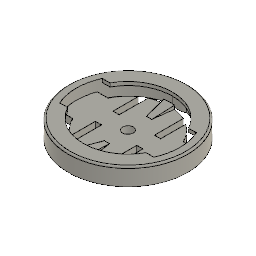
Blendr_Garmin_mount (Autodesk Fusion 360 design; units mm, degrees)
Autodesk Fusion 360 part; units mm, degrees
sketch "Sketch1" plane through (0, 0, 0) normal (0, 0, 1) x (1, 0, 0)
  circle A0 centre (0, 0) radius 1.5
  circle A1 centre (0, 0) radius 16.9
  circle A2 centre (0, 0) radius 14.6
  line L0 (0, 0) -> (25.4189, 0) construction
  line L1 (-6.75, -9.6177) -> (-6.75, 9.6177) construction
  line L2 (6.75, 9.6177) -> (6.75, -10.6368) construction
  line L3 (-6.75, 9.6177) -> (-6.75, 5)
  line L4 (6.75, 5) -> (6.75, 9.6177)
  line L5 (-6.75, -9.6177) -> (-6.75, -5)
  line L6 (6.75, -9.6177) -> (6.75, -5)
  line L7 (-10.6331, 5) -> (-13.7171, 5)
  line L8 (-13.7171, -5) -> (-10.6331, -5)
  arc A3 (-5, -10.6331) -> (5, -10.6331) centre (0, 0) ccw
  line L9 (13.7171, 5) -> (10.6331, 5)
  line L10 (10.6331, -5) -> (13.7171, -5)
  arc A4 (6.75, -9.6177) -> (10.6331, -5) centre (0, 0) ccw
  arc A5 (-6.75, 9.6177) -> (-10.6331, 5) centre (0, 0) ccw
  arc A6 (-10.6331, -5) -> (-6.75, -9.6177) centre (0, 0) ccw
  line L11 (-13.3404, 6) -> (-13.3404, -6) construction
  line L12 (13.3404, -6) -> (13.3404, 6) construction
  line L13 (-11.0797, 6) -> (-13.3404, 6)
  line L14 (11.0797, 6) -> (13.3404, 6)
  line L15 (13.3101, -6) -> (11.0797, -6)
  line L16 (-13.3101, -6) -> (-11.0797, -6)
  line L17 (-13.3404, -6) -> (-11.0797, -6) construction
  line L18 (-11.0797, 6) -> (-13.3404, 6) construction
  arc A7 (11.0797, 6) -> (-11.0797, 6) centre (0, 0) ccw
  line L19 (13.3404, 6) -> (11.0797, 6) construction
  line L20 (10.1026, 6) -> (-10.1026, 6) construction
  arc A8 (-11.0797, -6) -> (11.0797, -6) centre (0, 0) ccw
  line L21 (-10.1026, -6) -> (10.1026, -6) construction
  line L22 (11.0797, -6) -> (13.3404, -6) construction
  arc A9 (10.6331, 5) -> (6.75, 9.6177) centre (0, 0) ccw
  arc A10 (5, 10.6331) -> (-5, 10.6331) centre (0, 0) ccw
  line L23 (-5, -10.6368) -> (-5, -5)
  line L24 (-5, 5) -> (-5, 10.6368)
  line L25 (5, 10.6368) -> (5, 5)
  line L26 (5, -5) -> (5, -10.6368)
  line L27 (-5, 5) -> (-5, 2.5)
  line L28 (-5, 2.5) -> (-6.75, 2.5)
  line L29 (-6.75, 2.5) -> (-6.75, 5)
  line L30 (-5, -5) -> (-5, -2.5)
  line L31 (-5, -2.5) -> (-6.75, -2.5)
  line L32 (-6.75, -2.5) -> (-6.75, -5)
  line L33 (6.75, -5) -> (6.75, -2.5)
  line L34 (6.75, -2.5) -> (5, -2.5)
  line L35 (5, -2.5) -> (5, -5)
  line L36 (6.75, 5) -> (6.75, 2.5)
  line L37 (6.75, 2.5) -> (5, 2.5)
  line L38 (5, 2.5) -> (5, 5)
  line L39 (1.5, -11.75) -> (-1.5, -11.75) construction
  line L40 (-1.5, -11.75) -> (-1.5, 11.75) construction
  line L41 (-1.5, 11.75) -> (1.5, 11.75) construction
  line L42 (1.5, 11.75) -> (1.5, -11.75) construction
  line L43 (1.5, -11.75) -> (-1.5, 11.75) construction
  line L44 (-1.5, -11.75) -> (1.5, 11.75) construction
  arc A11 (-0.7598, -5.9517) -> (0.7598, -5.9517) centre (0, 0) ccw
  line L45 (-0.7598, -5.9517) -> (-1.4879, -11.6554)
  line L46 (0.7598, -5.9517) -> (1.5, -11.75)
  arc A12 (0.7598, 5.9517) -> (-0.7598, 5.9517) centre (0, 0) ccw
  line L47 (-0.7598, 5.9517) -> (-1.4879, 11.6554)
  line L48 (1.5, 11.6539) -> (0.7598, 5.9517)
  line L49 (0, 0) -> (0, 17.8654) construction
  line L50 (0, 0) -> (0, -17.7378) construction
  arc A13 (1.9907, -14.4637) -> (-1.9907, -14.4637) centre (0, -18.52) ccw
  arc A14 (-2.0011, 14.4622) -> (2.0011, 14.4622) centre (0, 18.5154) ccw
  dimension "d1" = 3
  dimension "d2" = 23.5
  dimension "d4" = 33.8
  dimension "d5" = 29.2
  dimension "d10" = 12
  dimension "d11" = 2.5
  dimension "d12" = 2.5
  dimension "d13" = 2.5
  dimension "d14" = 2.5
  dimension "d15" = 3
  dimension "d16" = 23.5
  dimension "d18" = 6
  dimension "d19" = 6
  constraint coincident A0.centre A1.centre
  constraint concentric A2 A5
  constraint horizontal L0
  constraint horizontal L9
  constraint parallel L8 L9
  constraint parallel L23 L25
  constraint parallel L1 L2
  constraint coincident L1 L3.end
  constraint coincident L2 L4.start
  constraint coincident L4.start L9
  constraint coincident L2.start A5
  constraint coincident L5.end L8
  constraint coincident L1 L5.end
  constraint coincident L6.start A5
  constraint coincident L2 L6.start
  constraint coincident L2 L6.end
  constraint coincident L6.end L8
  constraint coincident A10.end L23
  constraint collinear L7 L9
  constraint coincident L8.end A5
  constraint coincident A3.start L23
  constraint concentric A3 A5
  constraint coincident A3.end L25
  constraint concentric A3 A4
  constraint coincident L9.end A4
  constraint concentric A4 A9
  constraint concentric A5 A6
  constraint horizontal L19
  constraint perpendicular L11 L19
  constraint parallel L17 L19
  constraint parallel L11 L12
  constraint coincident L13.start L19
  constraint coincident L15.start L17
  constraint coincident A2 L15.start
  constraint coincident L15.end L17
  constraint coincident A2 L16.start
  constraint coincident L16.start L17
  constraint coincident A6 L21.start
  constraint collinear L17 L21
  constraint coincident A5 L20.end
  constraint collinear L18 L19
  constraint coincident L20.start A9
  constraint collinear L19 L20
  constraint coincident A4 L21.end
  constraint collinear L21 L22
  constraint coincident A10.start L25
  constraint concentric A9 A10
  constraint collinear L23 L24
  constraint collinear L25 L26
  constraint vertical L27
  constraint horizontal L28
  constraint vertical L29
  constraint vertical L30
  constraint horizontal L31
  constraint vertical L32
  constraint vertical L33
  constraint horizontal L34
  constraint vertical L35
  constraint vertical L36
  constraint horizontal L37
  constraint vertical L38
  constraint horizontal L39
  constraint perpendicular L39 L40
  constraint parallel L39 L41
  constraint parallel L40 L42
  constraint coincident L43 A0.centre
  constraint coincident L44 A0.centre
  constraint coincident L44 A11.start
  constraint coincident A3 L45.end
  constraint coincident L44 L45.end
  constraint parallel L43 L46
  constraint coincident L43 A12.end
  constraint coincident A10 L47.end
  constraint coincident L43 L47.end
  constraint coincident A10 L48.start
  constraint coincident L42 L48.start
  constraint coincident A2 L9.start
  constraint coincident A2 L10.end
  constraint coincident A2 L7.end
  constraint coincident A2 L8.start
  constraint vertical L49
  constraint vertical L50
  constraint coincident A2 A13.end
  constraint coincident A2 A13.start
  constraint coincident A2 A14.start
  constraint coincident A2 A14.end
  measures "d1" diameter of A0
  measures "d2" diameter of A5
  measures "d4" diameter of A1
  measures "d5" diameter of A2
  measures "d10" distance of L11.start L11.end
  measures "d11" distance of L3.end L28.end
  measures "d12" distance of L5.end L31.end
  measures "d13" distance of L26.start L34.end
  measures "d14" distance of L25.end L37.end
  measures "d15" distance of L40.end L41.end
  measures "d16" distance of L39.end L40.end
  measures "d18" radius of A11
  measures "d19" radius of A12
extrude "Extrude1" add sketch "Sketch1" along normal blind 2 contours A2 L3 L4 L5 L6 L7 L8 A3 L9 L10 A4 A5 A6 A9 A10 L23 L24 L25 L26 L27 L28 L29 L30 L31 L32 L33 L34 L35 L36 L37 L38 A11 L45 L46 A12 L47 L48
extrude "Extrude2" add sketch "Sketch1" along normal blind 3 contours A10 A12 L47 L48
chamfer "Chamfer1" distance 5.75 distance2 1 1 edges at (0, 6, 3) measured on face at (0.9217, 9.7816, 3)
extrude "Extrude3" add sketch "Sketch1" along normal blind 3 contours A3 A11 L45 L46
chamfer "Chamfer2" distance 5.75 distance2 1 1 edges at (0, -6, 3) measured on face at (-0.7463, -9.7965, 3)
extrude "Extrude4" add sketch "Sketch1" along normal blind 5 contours A1 | A2 A14 | A2 A13
extrude "Extrude5" add sketch "Sketch1" along normal blind 5 contours A2 L13 L14 A7 A14 | A2 L15 L16 A8 A13
extrude "Extrude6" cut sketch "Sketch1" along normal blind 4 contours A2 L13 L14 A7 A14 | A2 L15 L16 A8 A13
fillet "Fillet1" radius 0.5 1 edges at (-15.7563, -6.1113, 5)
component "Holder" placed x (1, 0, 0) y (0, 1, 0) z (0, 0, 1) at (0, 0, 0)
component "stem" placed x (1, 0, 0) y (0, 1, 0) z (0, 0, 1) at (0, 0, 0)
